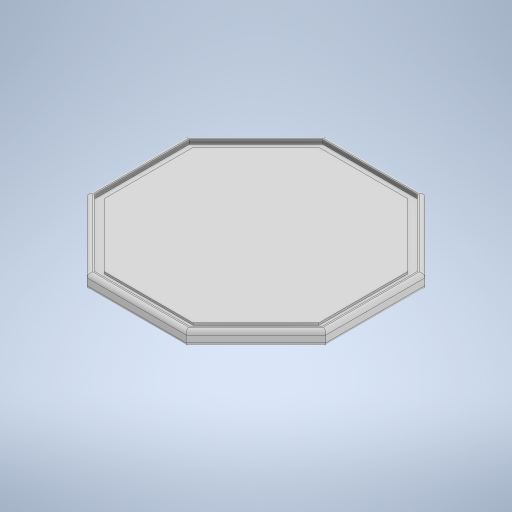
# Autodesk Inventor part: OV-PAM_bottom_2
Saved by Autodesk Inventor 2024 (Build 280153000, 153)
## iProperties
Created: 2023-06-16
Part Number: OV-PAM_bottom_2
Material: 일반
Document SubType Name: Modeling
Designer: jsw
Density: 1 g/cm^3
Appearance: 기본값
Author: jsw
Autodesk Inventor part; units mm, degrees
ref_plane "YZ Plane" through (0, 0, 0) normal (1, 0, 0) x (0, 1, 0)
ref_plane "XZ Plane" through (0, 0, 0) normal (0, 1, 0) x (-1, 0, 0)
ref_plane "XY Plane" through (0, 0, 0) normal (0, 0, 1) x (1, 0, 0)
sketch "스케치3" plane through (0, 0, 0) normal (0, 1, 0) x (-1, 0, 0)
  line L0 (35.7919, -14.8255) -> (14.8255, -35.7919)
  line L1 (14.8255, -35.7919) -> (-14.8255, -35.7919)
  line L2 (-14.8255, -35.7919) -> (-35.7919, -14.8255)
  line L3 (-35.7919, -14.8255) -> (-35.7919, 14.8255)
  line L4 (-35.7919, 14.8255) -> (-14.8255, 35.7919)
  line L5 (-14.8255, 35.7919) -> (14.8255, 35.7919)
  line L6 (14.8255, 35.7919) -> (35.7919, 14.8255)
  line L7 (35.7919, 14.8255) -> (35.7919, -14.8255)
  line L8 (13.5, -32.5919) -> (-13.5, -32.5919)
  line L9 (-13.5, -32.5919) -> (-32.5919, -13.5)
  line L10 (-32.5919, -13.5) -> (-32.5919, 13.5)
  line L11 (-32.5919, 13.5) -> (-13.5, 32.5919)
  line L12 (-13.5, 32.5919) -> (13.5, 32.5919)
  line L13 (13.5, 32.5919) -> (32.5919, 13.5)
  line L14 (32.5919, 13.5) -> (32.5919, -13.5)
  line L15 (32.5919, -13.5) -> (13.5, -32.5919)
  point P0 (0, 0)
  point P1 (0, 0)
  point P2 (0, 0)
  point P3 (0, 0)
  dimension "d66" = 27
  dimension "d67" = 3.2
  constraints: 32 end point, 3 coincident, 2 horizontal, 34 other
  measures "d66" distance of L8.start L8.end
  measures "d67" distance between parallel lines of L15 L0
extrude "돌출2" add sketch "스케치3" along normal blind 4.4 contours L0 L1 L2 L3 L4 L5 L6 L7 | L8 L9 L10 L11 L12 L13 L14 L15
sketch "스케치4" plane through (0, 4.4, 0) normal (0, 1, 0) x (1, 0, 0)
  line L0 (13.5, -32.5919) -> (-13.5, -32.5919)
  line L1 (-13.5, -32.5919) -> (-32.5919, -13.5)
  line L2 (-32.5919, -13.5) -> (-32.5919, 13.5)
  line L3 (-32.5919, 13.5) -> (-13.5, 32.5919)
  line L4 (-13.5, 32.5919) -> (13.5, 32.5919)
  line L5 (13.5, 32.5919) -> (32.5919, 13.5)
  line L6 (32.5919, 13.5) -> (32.5919, -13.5)
  line L7 (32.5919, -13.5) -> (13.5, -32.5919)
  line L8 (-14.1627, 34.1919) -> (14.1627, 34.1919)
  line L9 (14.1627, 34.1919) -> (34.1919, 14.1627)
  line L10 (34.1919, 14.1627) -> (34.1919, -14.1627)
  line L11 (34.1919, -14.1627) -> (14.1627, -34.1919)
  line L12 (14.1627, -34.1919) -> (-14.1627, -34.1919)
  line L13 (-14.1627, -34.1919) -> (-34.1919, -14.1627)
  line L14 (-34.1919, -14.1627) -> (-34.1919, 14.1627)
  line L15 (-34.1919, 14.1627) -> (-14.1627, 34.1919)
  line L16 (-13.3343, 32.1919) -> (13.3343, 32.1919)
  line L17 (13.3343, 32.1919) -> (32.1919, 13.3343)
  line L18 (32.1919, 13.3343) -> (32.1919, -13.3343)
  line L19 (32.1919, -13.3343) -> (13.3343, -32.1919)
  line L20 (13.3343, -32.1919) -> (-13.3343, -32.1919)
  line L21 (-13.3343, -32.1919) -> (-32.1919, -13.3343)
  line L22 (-32.1919, -13.3343) -> (-32.1919, 13.3343)
  line L23 (-32.1919, 13.3343) -> (-13.3343, 32.1919)
  line L24 (-14.8255, 35.7919) -> (-35.7919, 14.8255) projected
  point P0 (0, 0)
  point P1 (0, 0)
  point P2 (0, 0)
  point P3 (0, 0)
  dimension "d7" = 27
  dimension "d99" = 1.6
  dimension "d100" = 2
  constraints: 48 end point, 3 coincident, 3 horizontal, 51 other
  measures "d7" distance of L1.end L2.end
  measures "d99" distance between parallel lines of L15 L24
  measures "d100" distance between parallel lines of L23 L15
extrude "돌출3" cut sketch "스케치4" against normal blind 1.2 contours L0 L1 L2 L3 L4 L5 L6 L7 | L8 L9 L10 L11 L12 L13 L14 L15 | L16 L17 L18 L19 L20 L21 L22 L23
sketch "스케치11" plane through (0, 3.2, 0) normal (0, 1, 0) x (1, 0, 0)
  line L0 (-13.3343, 32.1919) -> (13.3343, 32.1919)
  line L1 (13.3343, 32.1919) -> (32.1919, 13.3343)
  line L2 (32.1919, 13.3343) -> (32.1919, -13.3343)
  line L3 (32.1919, -13.3343) -> (13.3343, -32.1919)
  line L4 (13.3343, -32.1919) -> (-13.3343, -32.1919)
  line L5 (-13.3343, -32.1919) -> (-32.1919, -13.3343)
  line L6 (-32.1919, -13.3343) -> (-32.1919, 13.3343)
  line L7 (-32.1919, 13.3343) -> (-13.3343, 32.1919)
  line L8 (-14.1627, 34.1919) -> (14.1627, 34.1919) projected
  line L9 (-12.0917, 29.1919) -> (12.0917, 29.1919)
  line L10 (12.0917, 29.1919) -> (29.1919, 12.0917)
  line L11 (29.1919, 12.0917) -> (29.1919, -12.0917)
  line L12 (29.1919, -12.0917) -> (12.0917, -29.1919)
  line L13 (12.0917, -29.1919) -> (-12.0917, -29.1919)
  line L14 (-12.0917, -29.1919) -> (-29.1919, -12.0917)
  line L15 (-29.1919, -12.0917) -> (-29.1919, 12.0917)
  line L16 (-29.1919, 12.0917) -> (-12.0917, 29.1919)
  point P0 (0, 0)
  point P1 (0, 0)
  point P2 (0, 0)
  dimension "d70" = 2
  dimension "d71" = 3
  constraints: 32 end point, 2 coincident, 2 horizontal, 34 other
  measures "d70" distance between parallel lines of L8 L0
  measures "d71" distance between parallel lines of L9 L0
extrude "돌출10" add sketch "스케치11" along normal blind 0.6 contours L0 L1 L2 L3 L4 L5 L6 L7 | L9 L10 L11 L12 L13 L14 L15 L16
fillet "모깎기1" radius 1.2 16 edges at (-25.3087, 4.4, 25.3087) (0, 4.4, 35.7919) (25.3087, 4.4, 25.3087) (35.7919, 4.4, 0) (25.3087, 4.4, -25.3087) (0, 4.4, -35.7919) (-25.3087, 4.4, -25.3087) (-35.7919, 4.4, 0) (-25.3087, 0, 25.3087) (0, 0, 35.7919) (25.3087, 0, 25.3087) (35.7919, 0, 0) (25.3087, 0, -25.3087) (0, 0, -35.7919) (-25.3087, 0, -25.3087) (-35.7919, 0, 0)
sketch "스케치12" plane through (0, 0, 0) normal (0, -1, 0) x (1, 0, 0)
  circle A0 centre (0, 0) radius 3.9688
  dimension "d101" = 7.9375
  constraints: 1 centre point, 1 coincident
  measures "d101" diameter of A0
extrude "돌출11" add sketch "스케치12" along normal blind 7.62
thread "스레드2" size "5/16-18 UNC" class "2A" standard "ANSI Unified Screw Threads" full length
